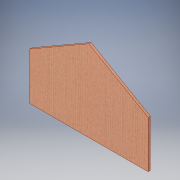
# Autodesk Inventor part: BA10
Saved by Autodesk Inventor 2017 (Build 210142000, 142)
## iProperties
Created: 2018-10-18
Part Number: BA10
Material: Wood (Oak)
Document SubType Name: Modeling
Designer: Dell
Density: 0.76 g/cm^3
Appearance: White Oak - Natural Medium Gloss
Author: Dell
Autodesk Inventor part; units mm, degrees
ref_plane "YZ Plane" through (0, 0, 0) normal (1, 0, 0) x (0, 1, 0)
ref_plane "XZ Plane" through (0, 0, 0) normal (0, 1, 0) x (-1, 0, 0)
ref_plane "XY Plane" through (0, 0, 0) normal (0, 0, 1) x (1, 0, 0)
sketch "Sketch1" plane through (0, 0, 0) normal (0, 0, 1) x (1, 0, 0)
  line L0 (0, 0) -> (505.9426, 0)
  line L1 (505.9426, 0) -> (505.9426, 203.2)
  line L2 (505.9426, 203.2) -> (0, 203.2)
  line L3 (0, 203.2) -> (0, 0)
  line L4 (0, 203.2) -> (252.9713, 349.253)
  line L5 (252.9713, 349.253) -> (505.9426, 203.2)
  point P0 (252.9713, 203.2)
  dimension "d0" = 505.9426
  dimension "d1" = 203.2
  dimension "d2" = 30
  constraints: 12 end point, 2 parallel, 1 horizontal, 1 midpoint, 1 perpendicular, 1 vertical alignment
  measures "d0" distance of L1.end L2.end
  measures "d1" distance of L0.end L1.end
  measures "d2" angle of L2 L5
extrude "Extrusion1" add sketch "Sketch1" along normal blind 10
sketch "Sketch2" plane through (0, 0, 10) normal (0, 0, 1) x (1, 0, 0)
  line L0 (0, 203.2) -> (0, 0) projected
  line L1 (252.9713, 349.253) -> (0, 203.2) projected
  line L2 (505.9426, 203.2) -> (252.9713, 349.253) projected
  line L3 (505.9426, 0) -> (505.9426, 203.2) projected
  line L4 (-10, 0) -> (-10, 208.9735)
  line L5 (-10, 208.9735) -> (252.9713, 360.8001)
  line L6 (252.9713, 360.8001) -> (515.9426, 208.9735)
  line L7 (515.9426, 208.9735) -> (515.9426, 0)
  line L8 (-10, 0) -> (0, 0)
  line L9 (0, 0) -> (505.9426, 0) projected
  line L10 (505.9426, 0) -> (515.9426, 0)
  dimension "d5" = 10
  constraints: 12 end point, 1 collinear, 1 horizontal, 3 other
  measures "d5" distance between parallel lines of L0 L4
extrude "Extrusion2" add sketch "Sketch2" against normal blind 10 contours L0 L8 L4 L5 L6 L7 L10 L3 L2 L1
body "Solid1"
